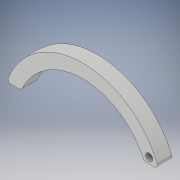
# Autodesk Inventor part: Flaschenhalterbügel
Saved by Autodesk Inventor 2019 (Build 230136000, 136)
## iProperties
Created: 2018-09-20
Part Number: Flaschenhalterbügel
Material: Generisch
Document SubType Name: Modeling
Designer: nico-
Density: 1 g/cm^3
Appearance: Vorgabe
Author: nico-
Autodesk Inventor part; units mm, degrees
ref_plane "YZ Plane" through (0, 0, 0) normal (1, 0, 0) x (0, 1, 0)
ref_plane "XZ Plane" through (0, 0, 0) normal (0, 1, 0) x (-1, 0, 0)
ref_plane "XY Plane" through (0, 0, 0) normal (0, 0, 1) x (1, 0, 0)
sketch "Skizze1" plane through (0, 0, 0) normal (0, 0, 1) x (1, 0, 0)
  line L0 (-52, 0) -> (-42, 0)
  line L1 (42, 0) -> (52, 0)
  arc A0 (52, 0) -> (-52, 0) centre (0, -17.9165) ccw
  arc A1 (42, 0) -> (-42, 0) centre (0, -17.9165) ccw
  circle A2 centre (45.5, 4) radius 2.5
  point P0 (0, 0)
  dimension "d2" = 55
  dimension "d3" = 5
  constraints: 4 end point, 4 point on circle, 3 centre point, 1 collinear, 1 concentric, 1 horizontal
  measures "d2" radius of A0
  measures "d3" diameter of A2
extrude "Extrusion1" add sketch "Skizze1" along normal blind 10
fillet "Rundung1" radius 2 4 edges at (52, 0, 5) (42, 0, 5) (-42, 0, 5) (-52, 0, 5)
